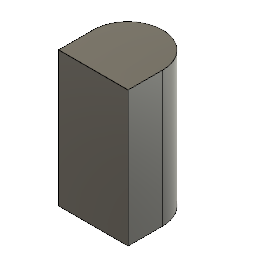
Rev B Battery Holder v100 (Autodesk Fusion 360 archive; units mm, degrees)
design "D Cell Holder"
Autodesk Fusion 360 part; units mm, degrees
sketch "Sketch1" plane through (0, 0, 0) normal (0, 0, 1) x (1, 0, 0)
sketch "Sketch2" plane through (0, 0, 0) normal (0, 1, 0) x (1, 0, 0)
  line L0 (-17.9997, 0.1117) -> (-17.9997, -17.8883)
  line L1 (-17.9997, -17.8883) -> (18.0003, -17.8883)
  line L2 (18.0003, -17.8883) -> (18, 0.0003)
  arc A0 (18, 0.0003) -> (-17.9997, -0.1117) centre (0, 0) ccw
  dimension "d2" = 18
  dimension "d3" = 36
  constraint vertical L0
  constraint perpendicular L0 L1
  constraint coincident L0 A0.end
  measures "d2" distance of L0.start L0.end
  measures "d3" distance of L0.end L1.end
extrude "Extrude1" add sketch "Sketch2" along normal blind 70
